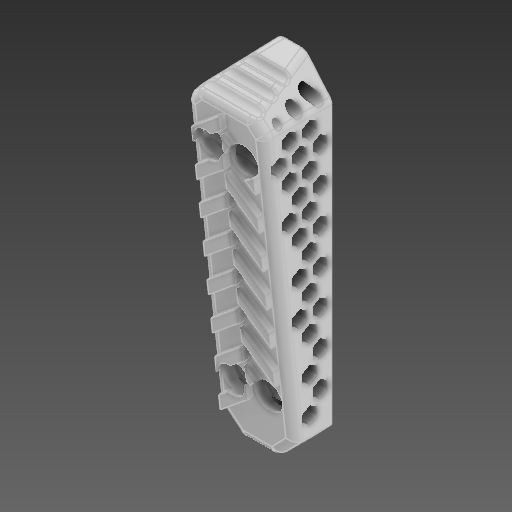
# Autodesk Inventor part: StockBack
Saved by Autodesk Inventor 2020.4 (Build 244396010, 396A)
## iProperties
Created: 2022-09-17
Part Number: StockBack
Material: Generic
Document SubType Name: Modeling
Designer: Val
Density: 1 g/cm^3
Appearance: Default
Author: Val
Autodesk Inventor part; units mm, degrees
ref_plane "YZ Plane" through (0, 0, 0) normal (1, 0, 0) x (0, 1, 0)
ref_plane "XZ Plane" through (0, 0, 0) normal (0, 1, 0) x (-1, 0, 0)
ref_plane "XY Plane" through (0, 0, 0) normal (0, 0, 1) x (1, 0, 0)
sketch "Base" plane through (0, 0, 0) normal (0, 0, 1) x (1, 0, 0)
  line L0 (0, 119.907465) -> (0, 0) construction
  line L1 (6.622372, 0) -> (0, 0)
  line L2 (14.2875, 7.953583) -> (6.622372, 0)
  line L3 (14.2875, 110.888748) -> (14.2875, 7.953583)
  line L4 (6.622372, 119.907465) -> (14.2875, 110.888748)
  line L5 (0, 119.907465) -> (6.622372, 119.907465)
  line L6 (0, 119.907465) -> (0, 0) construction
  line L7 (0, 119.907465) -> (-6.622372, 119.907465)
  line L8 (-6.622372, 119.907465) -> (-14.2875, 110.888748)
  line L9 (-14.2875, 110.888748) -> (-14.2875, 7.953583)
  line L10 (-14.2875, 7.953583) -> (-6.622372, 0)
  line L11 (-6.622372, 0) -> (0, 0)
  dimension "d0" = 136.058
  dimension "d1" = 139.638
  dimension "d2" = 90
  dimension "d3" = 40.3617
  dimension "d4" = 90
  dimension "d5" = 43.9419
  dimension "d6" = 14.2875
  dimension "d7" = 28.575
  dimension "d8" = 119.90746
  dimension "d9" = 14.2875
  dimension "d10" = 4.76839
  dimension "d11" = 82.69935
  dimension "d12" = 0
  dimension "d13" = 82.69935
  dimension "d14" = 4.76839
  constraints: 24 end point, 3 parallel, 1 horizontal, 1 vertical
  measures "d0" angle of L2 L3
  measures "d1" angle of L3 L4
  measures "d2" angle of L3 L7
  measures "d3" angle of L3 L8
  measures "d4" angle of L3 L11
  measures "d5" angle of L3 L10
  measures "d6" distance between parallel lines of L0 L3
  measures "d7" distance between parallel lines of L3 L9
  measures "d8" distance between parallel lines of L1 L5
  measures "d9" distance from line of point (0, 0) L3
  measures "d10" distance from line of point (0, 0) L2
  measures "d11" distance from line of point (0, 0) L4
  measures "d12" distance from line of point (0, 0) L1
  measures "d13" distance from line of point (0, 0) L8
  measures "d14" distance from line of point (0, 0) L10
extrude "BaseFeature" add sketch "Base" along normal blind 25.4
move faces "Move2" translate (0, 3.175, 0) faces at (-2.207457, 119.907465, 16.933333) (4.414915, 119.907465, 8.466667)
sketch "StockShapeProfile" plane through (-14.2875, 7.953583, 0) normal (-1, 0, 0) x (0, 0, 1)
  line L0 (-123.67713, 148.616895) -> (-186.350288, 165.971868)
  line L1 (-123.67713, 148.616895) -> (25.4, 107.335592)
  line L2 (-123.67713, 148.616895) -> (25.4, 148.616895)
  line L3 (25.4, 107.335592) -> (25.4, 148.616895)
  line L4 (25.4, 102.935165) -> (25.4, 0)
  point P0 (0, -7.953583)
  constraints: 6 end point, 2 collinear, 1 horizontal, 1 perpendicular
extrude "StockShapeFeature" cut sketch "StockShapeProfile" against normal through all both and the other way through all
sketch "StockProfile" plane through (-14.2875, 7.953583, 0) normal (-1, 0, 0) x (0, 0, 1)
  line L0 (25.4, 107.335592) -> (25.4, 102.935165)
  line L1 (25.4, 107.335592) -> (12.7, -7.953583)
  line L2 (0, -7.953583) -> (25.4, -7.953583)
  line L3 (25.4, 0) -> (25.4, -7.953583)
  line L4 (12.7, -7.953583) -> (25.4, -7.953583)
  line L5 (25.4, -7.953583) -> (25.4, 107.335592)
  constraints: 6 end point, 1 horizontal, 1 midpoint, 1 perpendicular
extrude "StockProfieFeature" cut sketch "StockProfile" against normal through all
fillet "StockFilletsFeature" radius 3.175 16 edges at (-14.2875, 110.8887, 12.4576) (-7.5586, 118.806, 12.7) (7.5586, 118.806, 12.7) (-14.2875, 7.9536, 6.7881) (-14.2875, 59.4212, 19.2457) (-12.4175, 113.089, 25.1576) (0, 115.2892, 25.4) (-10.4549, 3.9768, 13.1381) (10.4549, 3.9768, 13.1381) (14.2875, 59.4212, 19.2457) (14.2875, 110.8887, 12.4576) (12.4175, 113.089, 25.1576) (-6.6224, 0, 6.35) (6.6224, 0, 6.35) (-3.3112, 0, 12.7) (3.3112, 0, 12.7)
sketch "StockHoneycomb" plane through (-14.2875, 7.953583, 0) normal (-1, 0, 0) x (0, 0, 1)
  line L0 (7.973357, 94.585165) -> (5.223726, 96.172665)
  line L1 (5.223726, 96.172665) -> (5.223726, 99.347665)
  line L2 (5.223726, 99.347665) -> (7.973357, 100.935165)
  line L3 (7.973357, 100.935165) -> (10.722987, 99.347665)
  line L4 (10.722987, 99.347665) -> (10.722987, 96.172665)
  line L5 (10.722987, 96.172665) -> (7.973357, 94.585165)
  line L6 (0, 102.935165) -> (24.915259, 102.935165) construction
  line L7 (14.472618, 92.853114) -> (14.472618, 89.678114)
  line L8 (14.472618, 89.678114) -> (11.722987, 88.090614)
  line L9 (11.722987, 88.090614) -> (8.973357, 89.678114)
  line L10 (8.973357, 89.678114) -> (8.973357, 92.853114)
  line L11 (8.973357, 92.853114) -> (11.722987, 94.440614)
  line L12 (11.722987, 94.440614) -> (14.472618, 92.853114)
  line L13 (18.222249, 99.347665) -> (18.222249, 96.172665)
  line L14 (18.222249, 96.172665) -> (15.472618, 94.585165)
  line L15 (15.472618, 94.585165) -> (12.722987, 96.172665)
  line L16 (12.722987, 96.172665) -> (12.722987, 99.347665)
  line L17 (12.722987, 99.347665) -> (15.472618, 100.935165)
  line L18 (15.472618, 100.935165) -> (18.222249, 99.347665)
  line L19 (19.222249, 94.440614) -> (21.971879, 92.853114)
  line L20 (21.971879, 92.853114) -> (21.971879, 89.678114)
  line L21 (21.971879, 89.678114) -> (19.222249, 88.090614)
  line L22 (19.222249, 88.090614) -> (16.472618, 89.678114)
  line L23 (16.472618, 89.678114) -> (16.472618, 92.853114)
  line L24 (16.472618, 92.853114) -> (19.222249, 94.440614)
  line L25 (6.973357, 92.853114) -> (6.973357, 89.678114)
  line L26 (6.973357, 89.678114) -> (4.223726, 88.090614)
  line L27 (4.223726, 88.090614) -> (1.474095, 89.678114)
  line L28 (1.474095, 89.678114) -> (1.474095, 92.853114)
  line L29 (1.474095, 92.853114) -> (4.223726, 94.440614)
  line L30 (4.223726, 94.440614) -> (6.973357, 92.853114)
  line L31 (13.576149, 0) -> (24.915259, 102.935165)
  line L32 (10.722987, 99.347665) -> (12.722987, 99.347665) construction
  line L33 (4.223726, 91.265614) -> (19.222249, 91.265614) construction
  line L34 (7.973357, 87.946063) -> (5.223726, 86.358563)
  line L35 (5.223726, 86.358563) -> (5.223726, 83.183563)
  line L36 (5.223726, 83.183563) -> (7.973357, 81.596063)
  line L37 (7.973357, 81.596063) -> (10.722987, 83.183563)
  line L38 (10.722987, 83.183563) -> (10.722987, 86.358563)
  line L39 (10.722987, 86.358563) -> (7.973357, 87.946063)
  line L40 (18.222249, 83.183563) -> (18.222249, 86.358563)
  line L41 (18.222249, 86.358563) -> (15.472618, 87.946063)
  line L42 (15.472618, 87.946063) -> (12.722987, 86.358563)
  line L43 (12.722987, 86.358563) -> (12.722987, 83.183563)
  line L44 (12.722987, 83.183563) -> (15.472618, 81.596063)
  line L45 (15.472618, 81.596063) -> (18.222249, 83.183563)
  line L46 (5.223726, 84.771063) -> (18.222249, 84.771063) construction
  line L47 (14.472618, 76.689012) -> (14.472618, 79.864012)
  line L48 (14.472618, 79.864012) -> (11.722987, 81.451512)
  line L49 (11.722987, 81.451512) -> (8.973357, 79.864012)
  line L50 (8.973357, 79.864012) -> (8.973357, 76.689012)
  line L51 (8.973357, 76.689012) -> (11.722987, 75.101512)
  line L52 (11.722987, 75.101512) -> (14.472618, 76.689012)
  line L53 (19.222249, 75.101512) -> (21.971879, 76.689012) construction
  line L54 (21.971879, 76.689012) -> (21.971879, 79.864012) construction
  line L55 (21.971879, 79.864012) -> (19.222249, 81.451512) construction
  line L56 (19.222249, 81.451512) -> (16.472618, 79.864012) construction
  line L57 (16.472618, 79.864012) -> (16.472618, 76.689012) construction
  line L58 (16.472618, 76.689012) -> (19.222249, 75.101512) construction
  line L59 (6.973357, 76.689012) -> (6.973357, 79.864012)
  line L60 (6.973357, 79.864012) -> (4.223726, 81.451512)
  line L61 (4.223726, 81.451512) -> (1.474095, 79.864012)
  line L62 (1.474095, 79.864012) -> (1.474095, 76.689012)
  line L63 (1.474095, 76.689012) -> (4.223726, 75.101512)
  line L64 (4.223726, 75.101512) -> (6.973357, 76.689012)
  line L65 (4.223726, 78.276512) -> (19.222249, 78.276512) construction
  line L66 (5.223726, 70.194461) -> (5.223726, 73.369461)
  line L67 (5.223726, 73.369461) -> (7.973357, 74.956961)
  line L68 (7.973357, 68.606961) -> (5.223726, 70.194461)
  line L69 (10.722987, 70.194461) -> (7.973357, 68.606961)
  line L70 (10.722987, 73.369461) -> (10.722987, 70.194461)
  line L71 (7.973357, 74.956961) -> (10.722987, 73.369461)
  line L72 (12.722987, 73.369461) -> (15.472618, 74.956961)
  line L73 (15.472618, 74.956961) -> (18.222249, 73.369461)
  line L74 (12.722987, 70.194461) -> (12.722987, 73.369461)
  line L75 (15.472618, 68.606961) -> (12.722987, 70.194461)
  line L76 (18.222249, 70.194461) -> (15.472618, 68.606961)
  line L77 (18.222249, 73.369461) -> (18.222249, 70.194461)
  line L78 (4.062771, 104.935165) -> (5.937229, 107.336226) construction
  line L79 (5.639257, 103.704436) -> (7.513714, 106.105497)
  line L80 (4.360743, 108.566955) -> (2.486286, 106.165893)
  arc A0 (2.486286, 106.165893) -> (5.639257, 103.704436) centre (4.062771, 104.935165) ccw
  arc A1 (7.513714, 106.105497) -> (4.360743, 108.566955) centre (5.937229, 107.336226) ccw
  line L81 (11.674639, 104.935165) -> (12.196064, 105.603077) construction
  line L82 (10.098154, 106.165893) -> (10.619579, 106.833806)
  line L83 (13.77255, 104.372348) -> (13.251125, 103.704436)
  arc A2 (10.098154, 106.165893) -> (13.251125, 103.704436) centre (11.674639, 104.935165) ccw
  arc A3 (13.77255, 104.372348) -> (10.619579, 106.833806) centre (12.196064, 105.603077) ccw
  line L84 (11.722987, 68.462411) -> (14.472618, 66.874911)
  line L85 (14.472618, 66.874911) -> (14.472618, 63.699911)
  line L86 (14.472618, 63.699911) -> (11.722987, 62.112411)
  line L87 (11.722987, 62.112411) -> (8.973357, 63.699911)
  line L88 (8.973357, 63.699911) -> (8.973357, 66.874911)
  line L89 (8.973357, 66.874911) -> (11.722987, 68.462411)
  line L90 (4.223726, 68.462411) -> (6.973357, 66.874911)
  line L91 (6.973357, 66.874911) -> (6.973357, 63.699911)
  line L92 (6.973357, 63.699911) -> (4.223726, 62.112411)
  line L93 (4.223726, 62.112411) -> (1.474095, 63.699911)
  line L94 (1.474095, 63.699911) -> (1.474095, 66.874911)
  line L95 (1.474095, 66.874911) -> (4.223726, 68.462411)
  line L96 (7.973357, 61.96786) -> (10.722987, 60.38036)
  line L97 (10.722987, 60.38036) -> (10.722987, 57.20536)
  line L98 (10.722987, 57.20536) -> (7.973357, 55.61786)
  line L99 (7.973357, 55.61786) -> (5.223726, 57.20536)
  line L100 (5.223726, 57.20536) -> (5.223726, 60.38036)
  line L101 (5.223726, 60.38036) -> (7.973357, 61.96786)
  line L102 (0, 113.130847) -> (21.948176, 107.053125) construction
  line L103 (0, 113.130847) -> (0, 103.82436)
  line L104 (19.286508, 104.935165) -> (19.439857, 105.131595) construction
  line L105 (0, 111.055582) -> (21.726336, 105.039291) construction
  line L106 (21.592502, 103.82436) -> (21.948176, 107.053125)
  circle A4 centre (18.870704, 104.355876) radius 1.420711
  point P0 (0, -7.953583)
  point P1 (7.973357, 97.760165)
  point P2 (11.722987, 91.265614)
  point P3 (15.472618, 97.760165)
  point P4 (18.222249, 71.781961)
  point P5 (5, 106.135695)
  point P6 (11.935352, 105.269121)
  point P7 (11.722987, 65.287411)
  point P8 (4.223726, 65.287411)
  point P9 (7.973357, 58.79286)
  point P10 (19.363182, 105.03338)
  dimension "d21" = 3.175
  dimension "d22" = 2
  dimension "d24" = 2
  dimension "d25" = 2
  dimension "d26" = 2
  dimension "d27" = 2
  dimension "d28" = 2
  dimension "d29" = 2
  dimension "d30" = 2
  dimension "d31" = 1.4741
  dimension "d44" = 2
  dimension "d45" = 2
  dimension "d46" = 2
  dimension "d47" = 2
  dimension "d48" = 2
  dimension "d49" = 2
  dimension "d70" = 2
  dimension "d71" = 2
  dimension "d72" = 5
  dimension "d116" = 2
  dimension "d117" = 6.93535
  dimension "d118" = 6.93535
  dimension "d119" = 10.72299
  dimension "d120" = 6
  dimension "d121" = 2.28284
  dimension "d122" = 2.3483
  constraints: 210 end point, 45 symmetric about line, 19 parallel, 14 tangent, 8 point on circle, 5 centre point, 5 midpoint, 2 point on line, 1 equal radius, 1 horizontal, 104 other
  measures "d21" distance of L1.end L2.end
  measures "d22" distance from line of L6 L2.end
  measures "d24" distance between parallel lines of L5 L11
  measures "d25" distance between parallel lines of L15 L12
  measures "d26" distance between parallel lines of L4 L16
  measures "d27" distance between parallel lines of L24 L14
  measures "d28" distance between parallel lines of L30 L0
  measures "d29" distance between parallel lines of L10 L25
  measures "d30" distance between parallel lines of L23 L7
  measures "d31" distance from line of L31 L20.end
  measures "d44" distance from line of L75 L84.end
  measures "d45" distance between parallel lines of L89 L69
  measures "d46" distance between parallel lines of L68 L90
  measures "d47" distance between parallel lines of L88 L91
  measures "d48" distance between parallel lines of L92 L101
  measures "d49" distance between parallel lines of L87 L96
  measures "d70" radius of A1
  measures "d71" distance between parallel lines of L82 L79
  measures "d72" distance from line of L103 point (5, 106.136)
  measures "d116" distance between parallel lines of L102 L105
  measures "d117" horizontal distance of point (11.935, 105.269) point (5, 106.136)
  measures "d118" horizontal distance of A4.centre point (11.935, 105.269)
  measures "d119" distance between parallel lines of L97 L103
  measures "d120" distance between parallel lines of L81 L104
  measures "d121" distance from line of L104.end L106
  measures "d122" distance from line of point (19.363, 105.033) L106
extrude "StockHoneycomb1Feature" cut sketch "StockHoneycomb" against normal through all
sketch "StockHoneycomp2" plane through (14.2875, 7.953583, 0) normal (1, 0, 0) x (0, 0, -1)
  line L0 (-1.474095, 53.885809) -> (-1.474095, 50.710809)
  line L1 (-1.474095, 50.710809) -> (-4.223726, 49.123309)
  line L2 (-4.223726, 49.123309) -> (-6.973357, 50.710809)
  line L3 (-6.973357, 50.710809) -> (-6.973357, 53.885809)
  line L4 (-6.973357, 53.885809) -> (-4.223726, 55.473309)
  line L5 (-4.223726, 55.473309) -> (-1.474095, 53.885809)
  line L6 (-8.973357, 53.885809) -> (-8.973357, 50.710809)
  line L7 (-8.973357, 50.710809) -> (-11.722987, 49.123309)
  line L8 (-11.722987, 49.123309) -> (-14.472618, 50.710809)
  line L9 (-14.472618, 50.710809) -> (-14.472618, 53.885809)
  line L10 (-14.472618, 53.885809) -> (-11.722987, 55.473309)
  line L11 (-11.722987, 55.473309) -> (-8.973357, 53.885809)
  line L12 (-5.223726, 57.20536) -> (-7.973357, 55.61786)
  line L13 (-7.973357, 55.61786) -> (-10.722987, 57.20536)
  line L14 (-8.973357, 53.885809) -> (-6.973357, 53.885809) construction
  line L15 (-7.973357, 48.978758) -> (-5.223726, 47.391258)
  line L16 (-5.223726, 47.391258) -> (-5.223726, 44.216258)
  line L17 (-5.223726, 44.216258) -> (-7.973357, 42.628758)
  line L18 (-7.973357, 42.628758) -> (-10.722987, 44.216258)
  line L19 (-10.722987, 44.216258) -> (-10.722987, 47.391258)
  line L20 (-10.722987, 47.391258) -> (-7.973357, 48.978758)
  line L21 (-4.223726, 42.484207) -> (-1.474095, 40.896707)
  line L22 (-1.474095, 40.896707) -> (-1.474095, 37.721707)
  line L23 (-1.474095, 37.721707) -> (-4.223726, 36.134207)
  line L24 (-4.223726, 36.134207) -> (-6.973357, 37.721707)
  line L25 (-6.973357, 37.721707) -> (-6.973357, 40.896707)
  line L26 (-6.973357, 40.896707) -> (-4.223726, 42.484207)
  line L27 (-8.973357, 40.896707) -> (-8.973357, 37.721707)
  line L28 (-8.973357, 37.721707) -> (-11.722987, 36.134207)
  line L29 (-11.722987, 36.134207) -> (-14.472618, 37.721707)
  line L30 (-14.472618, 37.721707) -> (-14.472618, 40.896707)
  line L31 (-14.472618, 40.896707) -> (-11.722987, 42.484207)
  line L32 (-11.722987, 42.484207) -> (-8.973357, 40.896707)
  line L33 (-8.973357, 40.896707) -> (-6.973357, 40.896707) construction
  line L34 (-7.973357, 35.989657) -> (-5.223726, 34.402157)
  line L35 (-5.223726, 34.402157) -> (-5.223726, 31.227157)
  line L36 (-5.223726, 31.227157) -> (-7.973357, 29.639657)
  line L37 (-7.973357, 29.639657) -> (-10.722987, 31.227157)
  line L38 (-10.722987, 31.227157) -> (-10.722987, 34.402157)
  line L39 (-10.722987, 34.402157) -> (-7.973357, 35.989657)
  line L40 (-4.223726, 29.495106) -> (-1.474095, 27.907606)
  line L41 (-1.474095, 27.907606) -> (-1.474095, 24.732606)
  line L42 (-1.474095, 24.732606) -> (-4.223726, 23.145106)
  line L43 (-4.223726, 23.145106) -> (-6.973357, 24.732606)
  line L44 (-6.973357, 24.732606) -> (-6.973357, 27.907606)
  line L45 (-6.973357, 27.907606) -> (-4.223726, 29.495106)
  line L46 (-10.722987, 21.413055) -> (-7.973357, 23.000555)
  line L47 (-7.973357, 23.000555) -> (-5.223726, 21.413055)
  line L48 (-5.223726, 21.413055) -> (-5.223726, 18.238055)
  line L49 (-5.223726, 18.238055) -> (-7.973357, 16.650555)
  line L50 (-7.973357, 16.650555) -> (-10.722987, 18.238055)
  line L51 (-10.722987, 18.238055) -> (-10.722987, 21.413055)
  line L52 (-7.973357, 29.639657) -> (-7.973357, 23.000555) construction
  line L53 (-4.223726, 16.506004) -> (-1.474095, 14.918504)
  line L54 (-1.474095, 14.918504) -> (-1.474095, 11.743504)
  line L55 (-1.474095, 11.743504) -> (-4.223726, 10.156004)
  line L56 (-4.223726, 10.156004) -> (-6.973357, 11.743504)
  line L57 (-6.973357, 11.743504) -> (-6.973357, 14.918504)
  line L58 (-6.973357, 14.918504) -> (-4.223726, 16.506004)
  line L59 (-4.223726, 23.145106) -> (-4.223726, 16.506004) construction
  line L60 (-5.223726, 8.423953) -> (-5.223726, 5.248953)
  line L61 (-5.223726, 5.248953) -> (-7.973357, 3.661453)
  line L62 (-7.973357, 3.661453) -> (-10.722987, 5.248953)
  line L63 (-10.722987, 5.248953) -> (-10.722987, 8.423953)
  line L64 (-10.722987, 8.423953) -> (-7.973357, 10.011453)
  line L65 (-7.973357, 10.011453) -> (-5.223726, 8.423953)
  line L66 (-7.973357, 16.650555) -> (-7.973357, 10.011453) construction
  point P0 (0, -7.953583)
  point P1 (-4.223726, 52.298309)
  point P2 (-11.722987, 52.298309)
  point P3 (-7.973357, 45.803758)
  point P4 (-4.223726, 39.309207)
  point P5 (-11.722987, 39.309207)
  point P6 (-7.973357, 32.814657)
  point P7 (-4.223726, 26.320106)
  point P8 (-7.973357, 19.825555)
  point P9 (-4.223726, 13.331004)
  point P10 (-7.973357, 6.836453)
  dimension "d42" = 5
  dimension "d74" = 50
  dimension "d75" = 50
  dimension "d76" = 1.5
  dimension "d79" = 13
  dimension "d84" = 1.5
  dimension "d87" = 13
  dimension "d52" = 2
  dimension "d53" = 2
  dimension "d54" = 2
  dimension "d55" = 2
  dimension "d56" = 2
  dimension "d57" = 2
  dimension "d58" = 2
  dimension "d59" = 2
  dimension "d60" = 2
  dimension "d61" = 2
  dimension "d62" = 2
  dimension "d63" = 2
  dimension "d64" = 1
  dimension "d65" = 2
  dimension "d66" = 2
  constraints: 130 end point, 22 parallel, 1 horizontal, 1 perpendicular, 1 vertical, 130 other
  measures "d52" distance between parallel lines of L12 L4
  measures "d53" distance between parallel lines of L13 L11
  measures "d54" distance between parallel lines of L3 L6
  measures "d55" distance between parallel lines of L7 L20
  measures "d56" distance between parallel lines of L2 L15
  measures "d57" distance between parallel lines of L17 L26
  measures "d58" distance between parallel lines of L18 L32
  measures "d59" distance between parallel lines of L25 L27
  measures "d60" distance between parallel lines of L24 L34
  measures "d61" distance between parallel lines of L28 L39
  measures "d62" distance between parallel lines of L45 L36
  measures "d63" distance between parallel lines of L43 L47
  measures "d64" distance between parallel lines of L52 L44
  measures "d65" distance between parallel lines of L49 L58
  measures "d66" distance between parallel lines of L56 L65
extrude "StockHoneycomb2Feature" cut sketch "StockHoneycomp2" against normal through all
sketch "Sketch5" plane through (-10.547518, 115.289176, 25.4) normal (0, -0.1094954, 0.9939873) x (1, 0, 0)
  line L0 (-3.739982, -107.984873) -> (-3.739982, -4.427046) construction
  line L1 (3.925146, -115.986568) -> (-3.739982, -107.984873) construction
  line L2 (17.16989, -115.986568) -> (3.925146, -115.986568) construction
  line L3 (24.835018, -107.984873) -> (17.16989, -115.986568) construction
  line L4 (-0.564982, -12.027021) -> (10.547518, -2.702527)
  line L5 (-0.564982, -12.027021) -> (-0.564982, -17.027021)
  line L6 (-0.564982, -17.027021) -> (10.547518, -7.702527)
  line L7 (10.547518, -7.702527) -> (10.547518, -2.702527)
  line L8 (-3.739982, -107.984873) -> (-3.739982, -4.427046) construction
  line L9 (2.179188, -2.702527) -> (18.915847, -2.702527)
  line L10 (-0.564982, -5.950823) -> (2.179188, -2.702527)
  line L11 (-0.564982, -107.045963) -> (-0.564982, -5.950823) construction
  line L12 (18.915847, -2.702527) -> (21.660018, -5.950823)
  line L13 (21.660018, -5.950823) -> (21.660018, -107.045963) construction
  line L14 (-2.13433, -3.118138) -> (23.229365, -3.118138)
  line L15 (10.547518, -3.118138) -> (10.547518, -117.37716) construction
  line L16 (10.547518, -9.202527) -> (10.547518, -14.202527)
  line L17 (10.547518, -9.202527) -> (21.660018, -18.527021)
  line L18 (21.660018, -18.527021) -> (21.660018, -23.527021)
  line L19 (21.660018, -23.527021) -> (10.547518, -14.202527)
  line L20 (-0.564982, -25.027021) -> (10.547518, -15.702527)
  line L21 (-0.564982, -30.027021) -> (10.547518, -20.702527)
  line L22 (-0.564982, -25.027021) -> (-0.564982, -30.027021)
  line L23 (10.547518, -20.702527) -> (10.547518, -15.702527)
  line L24 (-0.564982, -38.027021) -> (10.547518, -28.702527)
  line L25 (-0.564982, -43.027021) -> (10.547518, -33.702527)
  line L26 (-0.564982, -38.027021) -> (-0.564982, -43.027021)
  line L27 (10.547518, -33.702527) -> (10.547518, -28.702527)
  line L28 (-0.564982, -51.027021) -> (10.547518, -41.702527)
  line L29 (-0.564982, -56.027021) -> (10.547518, -46.702527)
  line L30 (-0.564982, -51.027021) -> (-0.564982, -56.027021)
  line L31 (10.547518, -46.702527) -> (10.547518, -41.702527)
  line L32 (-0.564982, -64.027021) -> (10.547518, -54.702527)
  line L33 (-0.564982, -69.027021) -> (10.547518, -59.702527)
  line L34 (-0.564982, -64.027021) -> (-0.564982, -69.027021)
  line L35 (10.547518, -59.702527) -> (10.547518, -54.702527)
  line L36 (-0.564982, -77.027021) -> (10.547518, -67.702527)
  line L37 (-0.564982, -82.027021) -> (10.547518, -72.702527)
  line L38 (-0.564982, -77.027021) -> (-0.564982, -82.027021)
  line L39 (10.547518, -72.702527) -> (10.547518, -67.702527)
  line L40 (-0.564982, -90.027021) -> (10.547518, -80.702527)
  line L41 (-0.564982, -95.027021) -> (10.547518, -85.702527)
  line L42 (-0.564982, -90.027021) -> (-0.564982, -95.027021)
  line L43 (10.547518, -85.702527) -> (10.547518, -80.702527)
  line L44 (-0.564982, -103.027021) -> (10.547518, -93.702527)
  line L45 (-0.564982, -108.027021) -> (10.547518, -98.702527)
  line L46 (-0.564982, -103.027021) -> (-0.564982, -108.027021)
  line L47 (10.547518, -98.702527) -> (10.547518, -93.702527)
  line L48 (10.547518, -22.202527) -> (21.660018, -31.527021)
  line L49 (10.547518, -22.202527) -> (10.547518, -27.202527)
  line L50 (21.660018, -36.527021) -> (10.547518, -27.202527)
  line L51 (21.660018, -31.527021) -> (21.660018, -36.527021)
  line L52 (10.547518, -35.202527) -> (21.660018, -44.527021)
  line L53 (10.547518, -35.202527) -> (10.547518, -40.202527)
  line L54 (21.660018, -49.527021) -> (10.547518, -40.202527)
  line L55 (21.660018, -44.527021) -> (21.660018, -49.527021)
  line L56 (10.547518, -48.202527) -> (21.660018, -57.527021)
  line L57 (10.547518, -48.202527) -> (10.547518, -53.202527)
  line L58 (21.660018, -62.527021) -> (10.547518, -53.202527)
  line L59 (21.660018, -57.527021) -> (21.660018, -62.527021)
  line L60 (10.547518, -61.202527) -> (21.660018, -70.527021)
  line L61 (10.547518, -61.202527) -> (10.547518, -66.202527)
  line L62 (21.660018, -75.527021) -> (10.547518, -66.202527)
  line L63 (21.660018, -70.527021) -> (21.660018, -75.527021)
  line L64 (10.547518, -74.202527) -> (21.660018, -83.527021)
  line L65 (10.547518, -74.202527) -> (10.547518, -79.202527)
  line L66 (21.660018, -88.527021) -> (10.547518, -79.202527)
  line L67 (21.660018, -83.527021) -> (21.660018, -88.527021)
  line L68 (10.547518, -87.202527) -> (21.660018, -96.527021)
  line L69 (10.547518, -87.202527) -> (10.547518, -92.202527)
  line L70 (21.660018, -101.527021) -> (10.547518, -92.202527)
  line L71 (21.660018, -96.527021) -> (21.660018, -101.527021)
  point P0 (10.547518, -3.118138)
  point P1 (10.052211, -3.118138)
  dimension "d42" = 5
  dimension "d74" = 50
  dimension "d75" = 50
  dimension "d76" = 1.5
  dimension "d79" = 13
  dimension "d84" = 1.5
  dimension "d87" = 13
  constraints: 122 end point, 6 vertical, 3 collinear, 3 equal length, 3 parallel, 2 midpoint, 104 other
  measures "d42" distance of L4.start L5.end
  measures "d74" angle of L11 L4
  measures "d75" angle of L13 L17
  measures "d76" distance of L6.end L16.start
  measures "d79" distance of L4.start L20.start
  measures "d84" distance of L20.end L16.end
  measures "d87" distance of L16.start L48.start
extrude "Extrusion6" add sketch "Sketch5" along normal blind 2 contours L4 L14 L7 L6 L5 | L17 L18 L19 L16 | L20 L23 L21 L22 | L24 L27 L25 L26 | L28 L31 L29 L30 | L32 L35 L33 L34 | L36 L39 L37 L38 | L40 L43 L41 L42 | L44 L47 L45 L46 | L48 L51 L50 L49 | L52 L55 L54 L53 | L56 L59 L58 L57 | L60 L63 L62 L61 | L64 L67 L66 L65 | L68 L71 L70 L69
sketch "Sketch7" plane through (-14.2875, 9.234496, 0) normal (-1, 0, 0) x (0, 0, 1)
  line L0 (22.795487, 106.775902) -> (0, 113.088254) construction
  circle A0 centre (10.322078, 111.066887) radius 2
  line L1 (8.290721, 110.672969) -> (0, 110.672969) construction
  line L2 (0, 111.849934) -> (21.948176, 105.772212) construction
  circle A1 centre (2.702078, 111.554131) radius 2
  line L3 (0, 109.554131) -> (5.869109, 109.554131) construction
  circle A2 centre (16.422017, 109.377739) radius 2
  line L4 (0, 111.849934) -> (21.948176, 105.772212) construction
  circle A3 centre (22.521956, 107.68859) radius 2
  line L5 (0, 111.849934) -> (21.948176, 105.772212) construction
  line L6 (10.322078, 111.066887) -> (22.521956, 107.68859) construction
  line L7 (2.702078, 111.554131) -> (10.322078, 111.066887) construction
  point P0 (0, -9.234496)
  point P1 (9.138031, 110.55782)
  point P2 (8.290721, 109.554131)
  point P3 (12.672406, 108.340788)
  point P4 (18.645636, 106.686727)
  dimension "d94" = 4
  dimension "d95" = 12.65898
  dimension "d96" = 7.62
  dimension "d97" = 168.181
  constraints: 4 centre point, 4 end point, 4 tangent, 3 equal radius, 1 coincident, 1 midpoint
  measures "d94" diameter of A0
  measures "d95" distance of L6.start L6.end
  measures "d96" horizontal distance of L7.start L6.start
  measures "d97" angle of L0 L7
extrude "Extrusion7" cut sketch "Sketch7" against normal through all contours A0 | A2 | A3
fillet "Fillet2" radius 1 25 edges at (-9.7411, 115.2625, 23.6366) (-10.8231, 114.9396, 22.2654) (-10.7875, 115.0068, 21.9492) (-9.7165, 116.0322, 20.7313) (-10.7874, 115.0069, 21.9483) (-10.7876, 115.0066, 21.9491) (0, 116.6342, 20.5429) (9.7165, 116.0322, 20.7313) (10.7874, 115.0069, 21.9483) (10.7876, 115.0066, 21.9491) (10.7875, 115.0068, 21.9492) (10.8231, 114.9396, 22.2654) (9.7423, 115.2622, 23.6361) (0, 115.4633, 23.889) (8.2974, 117.7099, 14.6372) (8.9262, 116.943, 17.5236) (0, 117.3465, 17.9705) (-8.9262, 116.943, 17.5236) (-8.2974, 117.7099, 14.6372) (0, 118.3233, 14.443) (-7.4906, 118.6321, 11.4237) (-6.8618, 119.399, 8.5372) (6.8618, 119.399, 8.5372) (7.4906, 118.6321, 11.4237) (0, 119.0356, 11.8706)
sketch "MountHoles" plane through (0, 0, 0) normal (0, 0, -1) x (-1, 0, 0)
  circle A0 centre (6, 99.587465) radius 3
  circle A1 centre (-6, 99.587465) radius 3
  circle A2 centre (6, 20.32) radius 3
  circle A3 centre (-6, 20.32) radius 3
  point P0 (0, 0)
extrude "Extrusion8" cut sketch "MountHoles" against normal blind 25.4
ref_plane "Work Plane1" through (-11.1125, 103.224974, 25.077083) normal (0, 0, -1) x (-1, 0, 0)
sketch "Sketch10" plane through (-11.1125, 103.224974, 25.077083) normal (0, 0, -1) x (-1, 0, 0)
  circle A0 centre (-17.1125, -82.904974) radius 3
  circle A1 centre (-5.1125, -82.904974) radius 3
  circle A2 centre (-17.1125, -3.637509) radius 3
  circle A3 centre (-5.1125, -3.637509) radius 3
  circle A4 centre (-17.1125, -82.904974) radius 5
  circle A5 centre (-5.1125, -82.904974) radius 5
  circle A6 centre (-5.1125, -3.637509) radius 5
  circle A7 centre (-17.1125, -3.637509) radius 5
  point P0 (-11.1125, -103.224974)
  dimension "d103" = 10
  dimension "d104" = 10
  dimension "d105" = 10
  dimension "d106" = 10
  constraints: 4 centre point, 4 coincident
  measures "d103" diameter of A4
  measures "d104" diameter of A5
  measures "d105" diameter of A6
  measures "d106" diameter of A7
ref_plane "Work Plane2" through (-8.36833, 113.04088, 21.128136) normal (0, -0.1094954, 0.9939873) x (1, 0, 0)
extrude "Extrusion9" cut sketch "Sketch10" along normal up to surface contours A0 | A1 | A2 | A3 | A4 | A5 | A6 | A7 surface through (-8.36833, 113.04088, 21.128136) normal (0, -0.1094954, 0.9939873)
extrude "Extrusion10" cut sketch "Sketch10" against normal through all contours A0 | A1 | A2 | A3 | A4 | A5 | A6 | A7
delete faces "Delete1" heal yes whole lump no faces at (11.1125, 17.6129, 15.310897) (10.855196, 17.038459, 16.589017) (10.344765, 14.903352, 15.34861)
equation "\"d84\" = d76"
equation "\"d103\" = d105"
equation "\"d104\" = d105"
equation "\"d106\" = d105"
body "Solid1"
